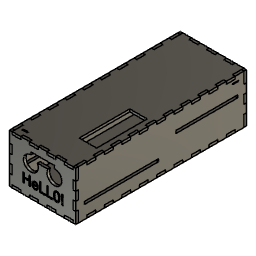
ShellV5 (Autodesk Fusion 360 design; units mm, degrees)
Autodesk Fusion 360 part; units mm, degrees
note: some values were not read from the file. Set by a fixed rule: which sketch regions a step uses.
(part 1 of 2)
sketch "Sketch1" plane through (0, 0, 0) normal (0, 0, 1) x (1, 0, 0)
  line L0 (0, 0) -> (-196, 0)
  line L1 (-196, 0) -> (-196, 76)
  line L2 (-196, 76) -> (0, 76)
  line L3 (0, 76) -> (0, 0)
  dimension "d7" = 196
  dimension "d8" = 76
  constraint horizontal L0
  constraint vertical L1
  constraint horizontal L2
  constraint vertical L3
  constraint coincident L0.start L3.end
  measures "d7" distance of L0.start L0.end
  measures "d8" distance of L0.start L2.end
extrude "Extrude1" add sketch "Sketch1" along normal blind 3 makes body 1
sketch "Sketch2" plane through (0, 0, 0) normal (1, 0, 0) x (0, 1, 0)
  line L0 (76, 0) -> (76, 56)
  line L1 (76, 56) -> (0, 56)
  line L2 (0, 56) -> (0, 0)
  line L3 (0, 56) -> (3, 56)
  line L4 (3, 56) -> (3, 53)
  line L5 (3, 53) -> (0, 53)
  line L6 (0, 53) -> (0, 56)
  line L7 (0, 53) -> (3, 53)
  line L8 (3, 53) -> (3, 43)
  line L9 (3, 43) -> (0, 43)
  line L10 (0, 43) -> (0, 53)
  line L11 (0, 43) -> (3, 43)
  line L12 (3, 43) -> (3, 33)
  line L13 (3, 33) -> (0, 33)
  line L14 (0, 33) -> (0, 43)
  line L15 (0, 33) -> (3, 33)
  line L16 (3, 33) -> (3, 23)
  line L17 (3, 23) -> (0, 23)
  line L18 (0, 23) -> (0, 33)
  line L19 (0, 23) -> (3, 23)
  line L20 (3, 23) -> (3, 13)
  line L21 (3, 13) -> (0, 13)
  line L22 (0, 13) -> (0, 23)
  line L23 (0, 13) -> (3, 13)
  line L24 (3, 13) -> (3, 3)
  line L25 (0, 3) -> (0, 13)
  line L26 (38, 0) -> (38, 56)
  line L27 (76, 13) -> (73, 13)
  line L28 (73, 53) -> (76, 53)
  line L29 (73, 56) -> (73, 53)
  line L30 (73, 23) -> (76, 23)
  line L31 (73, 43) -> (76, 43)
  line L32 (73, 23) -> (73, 13)
  line L33 (73, 13) -> (73, 3)
  line L34 (73, 33) -> (73, 23)
  line L35 (76, 56) -> (73, 56)
  line L36 (73, 53) -> (73, 43)
  line L37 (73, 33) -> (76, 33)
  line L38 (76, 53) -> (73, 53)
  line L39 (73, 13) -> (76, 13)
  line L40 (76, 43) -> (73, 43)
  line L41 (73, 43) -> (73, 33)
  line L42 (76, 23) -> (73, 23)
  line L43 (76, 33) -> (73, 33)
  line L44 (0, 56) -> (38, 56)
  line L45 (0, 56) -> (76, 56)
  line L46 (38, 28) -> (0, 28)
  line L47 (0, 3) -> (3, 3)
  line L48 (3, 3) -> (3, 0)
  line L49 (3, 0) -> (0, 0)
  line L50 (0, 0) -> (0, 3)
  line L51 (3, 3) -> (13, 3)
  line L52 (13, 3) -> (13, 0)
  line L53 (13, 0) -> (3, 0)
  line L54 (3, 0) -> (3, 3)
  line L55 (13, 3) -> (23, 3)
  line L56 (23, 3) -> (23, 0)
  line L57 (23, 0) -> (13, 0)
  line L58 (13, 0) -> (13, 3)
  line L59 (23, 3) -> (33, 3)
  line L60 (33, 3) -> (33, 0)
  line L61 (33, 0) -> (23, 0)
  line L62 (23, 0) -> (23, 3)
  line L63 (33, 3) -> (43, 3)
  line L64 (43, 3) -> (43, 0)
  line L65 (43, 0) -> (33, 0)
  line L66 (33, 0) -> (33, 3)
  line L67 (43, 0) -> (53, 0)
  line L68 (53, 0) -> (53, 3)
  line L69 (53, 3) -> (43, 3)
  line L70 (43, 3) -> (43, 0)
  line L71 (53, 3) -> (63, 3)
  line L72 (63, 3) -> (63, 0)
  line L73 (63, 0) -> (53, 0)
  line L74 (53, 0) -> (53, 3)
  line L75 (63, 3) -> (73, 3)
  line L76 (73, 3) -> (73, 0)
  line L77 (73, 0) -> (63, 0)
  line L78 (63, 0) -> (63, 3)
  line L79 (73, 3) -> (76, 3)
  line L80 (76, 3) -> (76, 0)
  line L81 (76, 0) -> (73, 0)
  line L82 (73, 0) -> (73, 3)
  line L83 (53, 56) -> (53, 53)
  line L84 (3, 53) -> (13, 53)
  line L85 (13, 56) -> (3, 56)
  line L86 (73, 53) -> (73, 56)
  line L87 (13, 56) -> (13, 53)
  line L88 (13, 53) -> (13, 56)
  line L89 (23, 56) -> (13, 56)
  line L90 (0, 53) -> (3, 53)
  line L91 (53, 56) -> (53, 53)
  line L92 (3, 56) -> (3, 53)
  line L93 (23, 56) -> (23, 53)
  line L94 (43, 53) -> (43, 56)
  line L95 (33, 56) -> (33, 53)
  line L96 (43, 53) -> (43, 56)
  line L97 (73, 56) -> (63, 56)
  line L98 (33, 53) -> (33, 56)
  line L99 (23, 53) -> (23, 56)
  line L100 (76, 53) -> (76, 56)
  line L101 (73, 56) -> (73, 53)
  line L102 (3, 53) -> (3, 56)
  line L103 (63, 53) -> (73, 53)
  line L104 (63, 53) -> (63, 56)
  line L105 (53, 53) -> (63, 53)
  line L106 (43, 56) -> (53, 56)
  line L107 (3, 56) -> (0, 56)
  line L108 (23, 53) -> (33, 53)
  line L109 (43, 56) -> (33, 56)
  line L110 (63, 56) -> (63, 53)
  line L111 (33, 56) -> (23, 56)
  line L112 (63, 56) -> (53, 56)
  line L113 (13, 53) -> (23, 53)
  line L114 (0, 56) -> (0, 53)
  line L115 (33, 53) -> (43, 53)
  line L116 (76, 56) -> (73, 56)
  line L117 (53, 53) -> (43, 53)
  line L118 (73, 53) -> (76, 53)
  point P0 (0, 56)
  point P1 (0, 56)
  point P2 (38, 56)
  point P3 (0, 56)
  point P4 (76, 56)
  dimension "d11" = 76
  dimension "d12" = 56
  dimension "d13" = 3
  dimension "d14" = 3
  dimension "d15" = 3
  dimension "d16" = 10
  dimension "d17" = 3
  dimension "d18" = 10
  dimension "d19" = 3
  dimension "d20" = 10
  dimension "d21" = 3
  dimension "d22" = 10
  dimension "d23" = 3
  dimension "d24" = 10
  dimension "d47" = 38
  dimension "d48" = 56
  dimension "d49" = 3
  dimension "d50" = 3
  dimension "d51" = 10
  dimension "d52" = 3
  dimension "d53" = 10
  dimension "d54" = 3
  dimension "d55" = 10
  dimension "d56" = 3
  dimension "d57" = 10
  dimension "d58" = 3
  dimension "d59" = 10
  dimension "d60" = 3
  dimension "d61" = 10
  dimension "d62" = 3
  dimension "d63" = 10
  dimension "d64" = 3
  dimension "d65" = 3
  dimension "d66" = 3
  constraint vertical L0
  constraint horizontal L1
  constraint vertical L2
  constraint coincident L2.end L49.end
  constraint horizontal L3
  constraint vertical L4
  constraint horizontal L5
  constraint vertical L6
  constraint horizontal L7
  constraint vertical L8
  constraint horizontal L9
  constraint vertical L10
  constraint horizontal L11
  constraint vertical L12
  constraint horizontal L13
  constraint vertical L14
  constraint horizontal L15
  constraint vertical L16
  constraint horizontal L17
  constraint vertical L18
  constraint horizontal L19
  constraint vertical L20
  constraint horizontal L21
  constraint vertical L22
  constraint horizontal L23
  constraint vertical L24
  constraint vertical L25
  constraint symmetric P3 L26 L0.end
  constraint symmetric L3.end L26 L29.start
  constraint symmetric L4.end L26 L28.start
  constraint symmetric L5.end L26 L28.end
  constraint symmetric L8.end L26 L31.start
  constraint symmetric L9.end L26 L31.end
  constraint symmetric L12.end L26 L34.start
  constraint symmetric L13.end L26 L37.end
  constraint symmetric L16.end L26 L30.start
  constraint symmetric L17.end L26 L30.end
  constraint symmetric L20.end L26 L27.end
  constraint symmetric L21.end L26 L27.start
  constraint symmetric L24.end L26 L33.end
  constraint midpoint L26 L46.start
  constraint midpoint L18 L46.end
  constraint horizontal L47
  constraint vertical L48
  constraint horizontal L49
  constraint vertical L50
  constraint horizontal L51
  constraint vertical L52
  constraint horizontal L53
  constraint vertical L54
  constraint horizontal L55
  constraint vertical L56
  constraint horizontal L57
  constraint vertical L58
  constraint horizontal L59
  constraint vertical L60
  constraint horizontal L61
  constraint vertical L62
  constraint horizontal L63
  constraint vertical L64
  constraint horizontal L65
  constraint vertical L66
  constraint horizontal L67
  constraint vertical L68
  constraint horizontal L69
  constraint vertical L70
  constraint horizontal L71
  constraint vertical L72
  constraint horizontal L73
  constraint vertical L74
  constraint horizontal L75
  constraint vertical L76
  constraint horizontal L77
  constraint vertical L78
  constraint horizontal L79
  constraint vertical L80
  constraint horizontal L81
  constraint vertical L82
  constraint symmetric L2.end L46 P3
  constraint symmetric L0.start L46 P4
  constraint symmetric L24.end L46 L4.end
  constraint symmetric L25.start L46 L5.end
  constraint symmetric L26.start L46 P2
  constraint symmetric L33.end L46 L28.start
  constraint symmetric L46 L24.end L4.end
  constraint symmetric L46 L48.end L3.end
  constraint symmetric L46 L2.end P3
  constraint symmetric L46 L51.end L84.end
  constraint symmetric L46 L52.end L85.start
  constraint symmetric L46 L55.end L93.end
  constraint symmetric L46 L56.end L89.start
  constraint symmetric L46 L59.end L95.end
  constraint symmetric L46 L60.end L95.start
  constraint symmetric L46 L63.end L94.start
  constraint symmetric L46 L64.end L94.end
  constraint symmetric L46 L67.end L83.start
  constraint symmetric L46 L68.end L83.end
  constraint symmetric L46 L71.end L103.start
  constraint symmetric L46 L72.end L97.end
  constraint symmetric L46 L33.end L28.start
  constraint symmetric L46 L76.end L29.start
  constraint symmetric L46 L79.end L28.end
  constraint symmetric L46 L0.start P4
  measures "d11" distance of L2.end L0.start
  measures "d12" distance of L2.end P3
  measures "d13" distance of P3 L3.end
  measures "d14" distance of P3 L5.end
  measures "d15" distance of L5.end L4.end
  measures "d16" distance of L5.end L9.end
  measures "d17" distance of L9.end L8.end
  measures "d18" distance of L9.end L13.end
  measures "d19" distance of L13.end L12.end
  measures "d20" distance of L13.end L17.end
  measures "d21" distance of L17.end L16.end
  measures "d22" distance of L17.end L21.end
  measures "d23" distance of L21.end L20.end
  measures "d24" distance of L21.end L25.start
  measures "d47" distance of L2.end L26.start
  measures "d48" distance of L26.start P2
  measures "d49" distance of L25.start L24.end
  measures "d50" distance of L25.start L2.end
  measures "d51" distance of L24.end L51.end
  measures "d52" distance of L24.end L48.end
  measures "d53" distance of L51.end L55.end
  measures "d54" distance of L51.end L52.end
  measures "d55" distance of L55.end L59.end
  measures "d56" distance of L55.end L56.end
  measures "d57" distance of L59.end L63.end
  measures "d58" distance of L59.end L60.end
  measures "d59" distance of L64.end L67.end
  measures "d60" distance of L64.end L63.end
  measures "d61" distance of L68.end L71.end
  measures "d62" distance of L68.end L67.end
  measures "d63" distance of L71.end L33.end
  measures "d64" distance of L71.end L72.end
  measures "d65" distance of L33.end L79.end
  measures "d66" distance of L33.end L76.end
extrude "Extrude2" add sketch "Sketch2" against normal blind 3 separate body contours L0 L76 L79 L80 L81 L82 | L0 L27 L33 L39 L79 | L26 L32 L33 L34 L36 L41 L63 L69 L71 L75 L103 L105 L115 L117 | L68 L71 L72 L73 L74 L78 | L0 L30 L34 L37 L42 L43 | L26 L63 L64 L65 L70 | L0 L28 L31 L36 L38 L40 L118 | L26 L60 L63 L65 L66 | L0 L1 L28 L29 L35 L38 L45 L86 L100 L101 L116 L118 | L16 L20 L24 L26 L46 L51 L55 L59 L63 | L8 L12 L16 L26 L46 L84 L108 L113 L115 | L52 L55 L56 L57 L58 L62 | L1 L45 L83 L91 L104 L105 L110 L112 | L1 L26 L44 L45 L95 L98 L109 L115 | L1 L26 L45 L94 L96 L109 L115 | L2 L13 L15 L16 L18 L46 | L2 L16 L17 L18 L19 L46 | L2 L47 L48 L49 L50 L54 | L1 L44 L45 L87 L88 L89 L93 L99 L113 | L2 L5 L7 L8 L9 L10 L11 L90 | L2 L21 L23 L24 L25 L47 | L1 L2 L3 L4 L5 L6 L7 L44 L45 L90 L92 L102 L107 L114 makes body 2
combine "Combine1" operation cut target body 1 tool bodies 2 keep tools
sketch "Sketch3" plane through (0, 76, 0) normal (0, 1, 0) x (-1, 0, 0)
  line L0 (3, 3) -> (3, 0)
  line L1 (3, 0) -> (196, 0)
  line L2 (196, 0) -> (196, 3)
  line L3 (196, 3) -> (3, 3)
  line L4 (0, 0) -> (196, 0)
  line L5 (196, 0) -> (196, 56)
  line L6 (196, 56) -> (0, 56)
  line L7 (0, 56) -> (0, 0)
  line L8 (0, 56) -> (3, 56)
  line L9 (3, 56) -> (3, 53)
  line L10 (3, 53) -> (0, 53)
  line L11 (0, 53) -> (0, 56)
  line L12 (0, 53) -> (3, 53)
  line L13 (3, 53) -> (3, 43)
  line L14 (3, 43) -> (0, 43)
  line L15 (0, 43) -> (0, 53)
  line L16 (0, 43) -> (3, 43)
  line L17 (3, 43) -> (3, 33)
  line L18 (3, 33) -> (0, 33)
  line L19 (0, 33) -> (0, 43)
  line L20 (0, 0) -> (3, 0)
  line L21 (3, 0) -> (3, 3)
  line L22 (3, 3) -> (0, 3)
  line L23 (0, 3) -> (0, 0)
  line L24 (0, 3) -> (3, 3)
  line L25 (3, 3) -> (3, 13)
  line L26 (3, 13) -> (0, 13)
  line L27 (0, 13) -> (0, 3)
  line L28 (0, 13) -> (3, 13)
  line L29 (3, 13) -> (3, 23)
  line L30 (3, 23) -> (0, 23)
  line L31 (0, 23) -> (0, 13)
  line L32 (3, 3) -> (13, 3)
  line L33 (13, 3) -> (13, 0)
  line L34 (13, 0) -> (3, 0)
  line L35 (3, 0) -> (3, 3)
  line L36 (13, 0) -> (23, 0)
  line L37 (23, 0) -> (23, 3)
  line L38 (23, 3) -> (13, 3)
  line L39 (13, 3) -> (13, 0)
  line L40 (23, 0) -> (33, 0)
  line L41 (33, 0) -> (33, 3)
  line L42 (33, 3) -> (23, 3)
  line L43 (23, 3) -> (23, 0)
  line L44 (33, 0) -> (43, 0)
  line L45 (43, 0) -> (43, 3)
  line L46 (43, 3) -> (33, 3)
  line L47 (33, 3) -> (33, 0)
  line L48 (43, 0) -> (53, 0)
  line L49 (53, 0) -> (53, 3)
  line L50 (53, 3) -> (43, 3)
  line L51 (43, 3) -> (43, 0)
  line L52 (53, 0) -> (63, 0)
  line L53 (63, 0) -> (63, 3)
  line L54 (63, 3) -> (53, 3)
  line L55 (53, 3) -> (53, 0)
  line L56 (63, 0) -> (73, 0)
  line L57 (73, 0) -> (73, 3)
  line L58 (73, 3) -> (63, 3)
  line L59 (63, 3) -> (63, 0)
  line L60 (73, 0) -> (83, 0)
  line L61 (83, 0) -> (83, 3)
  line L62 (83, 3) -> (73, 3)
  line L63 (73, 3) -> (73, 0)
  line L64 (83, 0) -> (93, 0)
  line L65 (93, 0) -> (93, 3)
  line L66 (93, 3) -> (83, 3)
  line L67 (83, 3) -> (83, 0)
  line L68 (93, 0) -> (103, 0)
  line L69 (103, 0) -> (103, 3)
  line L70 (103, 3) -> (93, 3)
  line L71 (93, 3) -> (93, 0)
  line L72 (103, 0) -> (113, 0)
  line L73 (113, 0) -> (113, 3)
  line L74 (113, 3) -> (103, 3)
  line L75 (103, 3) -> (103, 0)
  line L76 (113, 0) -> (123, 0)
  line L77 (123, 0) -> (123, 3)
  line L78 (123, 3) -> (113, 3)
  line L79 (113, 3) -> (113, 0)
  line L80 (123, 0) -> (133, 0)
  line L81 (133, 0) -> (133, 3)
  line L82 (133, 3) -> (123, 3)
  line L83 (123, 3) -> (123, 0)
  line L84 (133, 0) -> (143, 0)
  line L85 (143, 0) -> (143, 3)
  line L86 (143, 3) -> (133, 3)
  line L87 (133, 3) -> (133, 0)
  line L88 (143, 0) -> (153, 0)
  line L89 (153, 0) -> (153, 3)
  line L90 (153, 3) -> (143, 3)
  line L91 (143, 3) -> (143, 0)
  line L92 (153, 0) -> (163, 0)
  line L93 (163, 0) -> (163, 3)
  line L94 (163, 3) -> (153, 3)
  line L95 (153, 3) -> (153, 0)
  line L96 (163, 3) -> (173, 3)
  line L97 (173, 3) -> (173, 0)
  line L98 (173, 0) -> (163, 0)
  line L99 (163, 0) -> (163, 3)
  line L100 (173, 3) -> (183, 3)
  line L101 (183, 3) -> (183, 0)
  line L102 (183, 0) -> (173, 0)
  line L103 (173, 0) -> (173, 3)
  line L104 (183, 3) -> (193, 3)
  line L105 (193, 3) -> (193, 0)
  line L106 (193, 0) -> (183, 0)
  line L107 (183, 0) -> (183, 3)
  line L108 (193, 3) -> (196, 3)
  line L109 (196, 3) -> (196, 0)
  line L110 (196, 0) -> (193, 0)
  line L111 (193, 0) -> (193, 3)
  line L112 (0, 0) -> (78, 0)
  line L113 (0, 0) -> (88, 0)
  line L114 (88, 28) -> (196, 28)
  line L115 (3, 53) -> (3, 56)
  line L116 (153, 56) -> (163, 56)
  line L117 (163, 56) -> (163, 53)
  line L118 (133, 53) -> (133, 56)
  line L119 (133, 53) -> (123, 53)
  line L120 (173, 53) -> (183, 53)
  line L121 (193, 56) -> (193, 53)
  line L122 (3, 56) -> (196, 56)
  line L123 (196, 53) -> (3, 53)
  line L124 (196, 53) -> (196, 56)
  line L125 (173, 56) -> (173, 53)
  line L126 (143, 53) -> (133, 53)
  line L127 (183, 56) -> (183, 53)
  line L128 (193, 53) -> (196, 53)
  line L129 (196, 56) -> (196, 53)
  line L130 (193, 53) -> (193, 56)
  line L131 (183, 53) -> (193, 53)
  line L132 (123, 56) -> (133, 56)
  line L133 (153, 56) -> (153, 53)
  line L134 (33, 53) -> (33, 56)
  line L135 (173, 53) -> (173, 56)
  line L136 (0, 56) -> (196, 56)
  line L137 (163, 53) -> (173, 53)
  line L138 (163, 56) -> (163, 53)
  line L139 (53, 56) -> (53, 53)
  line L140 (93, 53) -> (93, 56)
  line L141 (183, 53) -> (183, 56)
  line L142 (143, 56) -> (153, 56)
  line L143 (113, 56) -> (123, 56)
  line L144 (183, 56) -> (173, 56)
  line L145 (103, 56) -> (113, 56)
  line L146 (143, 53) -> (143, 56)
  line L147 (196, 56) -> (193, 56)
  line L148 (0, 56) -> (78, 56)
  line L149 (63, 56) -> (73, 56)
  line L150 (0, 56) -> (88, 56)
  line L151 (133, 56) -> (133, 53)
  line L152 (73, 53) -> (63, 53)
  line L153 (13, 56) -> (3, 56)
  line L154 (83, 56) -> (83, 53)
  line L155 (153, 53) -> (143, 53)
  line L156 (133, 56) -> (143, 56)
  line L157 (0, 53) -> (3, 53)
  line L158 (123, 53) -> (113, 53)
  line L159 (93, 56) -> (93, 53)
  line L160 (103, 53) -> (93, 53)
  line L161 (73, 56) -> (83, 56)
  line L162 (13, 56) -> (23, 56)
  line L163 (153, 53) -> (153, 56)
  line L164 (83, 53) -> (83, 56)
  line L165 (163, 53) -> (153, 53)
  line L166 (143, 56) -> (143, 53)
  line L167 (13, 53) -> (13, 56)
  line L168 (123, 56) -> (123, 53)
  line L169 (173, 56) -> (163, 56)
  line L170 (53, 53) -> (43, 53)
  line L171 (83, 56) -> (93, 56)
  line L172 (43, 53) -> (33, 53)
  line L173 (103, 53) -> (103, 56)
  line L174 (193, 56) -> (183, 56)
  line L175 (113, 56) -> (113, 53)
  line L176 (33, 56) -> (33, 53)
  line L177 (23, 56) -> (33, 56)
  line L178 (113, 53) -> (103, 53)
  line L179 (0, 56) -> (3, 56)
  line L180 (23, 53) -> (23, 56)
  line L181 (73, 53) -> (73, 56)
  line L182 (103, 56) -> (103, 53)
  line L183 (93, 56) -> (103, 56)
  line L184 (3, 53) -> (13, 53)
  line L185 (73, 56) -> (73, 53)
  line L186 (63, 56) -> (63, 53)
  line L187 (3, 56) -> (3, 53)
  line L188 (53, 56) -> (63, 56)
  line L189 (33, 56) -> (43, 56)
  line L190 (113, 53) -> (113, 56)
  line L191 (53, 53) -> (53, 56)
  line L192 (43, 53) -> (43, 56)
  line L193 (63, 53) -> (53, 53)
  line L194 (63, 53) -> (63, 56)
  line L195 (123, 53) -> (123, 56)
  line L196 (93, 53) -> (83, 53)
  line L197 (33, 53) -> (23, 53)
  line L198 (13, 53) -> (13, 56)
  line L199 (43, 56) -> (53, 56)
  line L200 (0, 53) -> (0, 56)
  line L201 (83, 53) -> (73, 53)
  line L202 (23, 53) -> (13, 53)
  line L203 (3, 56) -> (3, 53)
  line L204 (43, 56) -> (43, 53)
  line L205 (23, 56) -> (23, 53)
  line L206 (3, 53) -> (0, 53)
  line L207 (196, 0) -> (98, 0)
  line L208 (98, 0) -> (98, 53)
  line L209 (0, 33) -> (3, 33)
  line L210 (3, 33) -> (3, 23)
  line L211 (3, 23) -> (0, 23)
  line L212 (0, 23) -> (0, 33)
  line L213 (193, 53) -> (193, 56)
  line L214 (196, 3) -> (193, 3)
  line L215 (193, 3) -> (196, 3)
  line L216 (193, 43) -> (193, 33)
  line L217 (196, 3) -> (196, 0)
  line L218 (193, 56) -> (193, 53)
  line L219 (193, 56) -> (193, 53)
  line L220 (196, 33) -> (196, 43)
  line L221 (196, 33) -> (193, 33)
  line L222 (193, 56) -> (193, 53)
  line L223 (196, 56) -> (193, 56)
  line L224 (196, 56) -> (193, 56)
  line L225 (196, 43) -> (193, 43)
  line L226 (196, 53) -> (196, 56)
  line L227 (196, 13) -> (193, 13)
  line L228 (193, 13) -> (196, 13)
  line L229 (193, 23) -> (196, 23)
  line L230 (196, 13) -> (196, 3)
  line L231 (193, 43) -> (196, 43)
  line L232 (196, 53) -> (196, 56)
  line L233 (196, 53) -> (193, 53)
  line L234 (196, 23) -> (196, 33)
  line L235 (196, 53) -> (193, 53)
  line L236 (193, 23) -> (196, 23)
  line L237 (196, 56) -> (196, 0)
  line L238 (193, 3) -> (193, 13)
  line L239 (193, 53) -> (196, 53)
  line L240 (193, 3) -> (193, 0)
  line L241 (193, 33) -> (193, 23)
  line L242 (193, 53) -> (193, 43)
  line L243 (193, 33) -> (196, 33)
  line L244 (196, 43) -> (196, 53)
  line L245 (196, 23) -> (196, 13)
  line L246 (193, 0) -> (193, 3)
  line L247 (196, 0) -> (193, 0)
  line L248 (193, 0) -> (193, 3)
  line L249 (193, 53) -> (196, 53)
  line L250 (193, 13) -> (193, 23)
  point P0 (0, 56)
  point P1 (196, 56)
  point P2 (196, 0)
  point P3 (196, 56)
  dimension "d69" = 196
  dimension "d70" = 56
  dimension "d71" = 3
  dimension "d72" = 3
  dimension "d73" = 3
  dimension "d74" = 10
  dimension "d75" = 3
  dimension "d76" = 10
  dimension "d77" = 3
  dimension "d78" = 3
  dimension "d79" = 3
  dimension "d80" = 10
  dimension "d81" = 3
  dimension "d82" = 10
  dimension "d83" = 10
  dimension "d84" = 3
  dimension "d85" = 10
  dimension "d86" = 3
  dimension "d87" = 10
  dimension "d88" = 3
  dimension "d89" = 10
  dimension "d90" = 3
  dimension "d91" = 10
  dimension "d92" = 3
  dimension "d93" = 10
  dimension "d94" = 3
  dimension "d95" = 10
  dimension "d96" = 3
  dimension "d97" = 10
  dimension "d98" = 3
  dimension "d99" = 10
  dimension "d100" = 3
  dimension "d101" = 10
  dimension "d102" = 3
  dimension "d103" = 10
  dimension "d104" = 10
  dimension "d105" = 3
  dimension "d106" = 10
  dimension "d107" = 3
  dimension "d108" = 10
  dimension "d109" = 3
  dimension "d110" = 10
  dimension "d111" = 3
  dimension "d112" = 10
  dimension "d113" = 3
  dimension "d114" = 10
  dimension "d115" = 3
  dimension "d116" = 10
  dimension "d117" = 3
  dimension "d118" = 10
  dimension "d119" = 3
  dimension "d120" = 3
  dimension "d121" = 3
  dimension "d122" = 98
  dimension "d123" = 3
  dimension "d124" = 10
  constraint horizontal L4
  constraint vertical L5
  constraint horizontal L6
  constraint vertical L7
  constraint coincident L4.start L7.end
  constraint horizontal L8
  constraint vertical L9
  constraint horizontal L10
  constraint vertical L11
  constraint horizontal L12
  constraint vertical L13
  constraint horizontal L14
  constraint vertical L15
  constraint horizontal L16
  constraint vertical L17
  constraint horizontal L18
  constraint vertical L19
  constraint horizontal L20
  constraint vertical L21
  constraint horizontal L22
  constraint vertical L23
  constraint horizontal L24
  constraint vertical L25
  constraint horizontal L26
  constraint vertical L27
  constraint horizontal L28
  constraint vertical L29
  constraint horizontal L30
  constraint vertical L31
  constraint horizontal L32
  constraint vertical L33
  constraint horizontal L34
  constraint vertical L35
  constraint horizontal L36
  constraint vertical L37
  constraint horizontal L38
  constraint vertical L39
  constraint horizontal L40
  constraint vertical L41
  constraint horizontal L42
  constraint vertical L43
  constraint horizontal L44
  constraint vertical L45
  constraint horizontal L46
  constraint vertical L47
  constraint horizontal L48
  constraint vertical L49
  constraint horizontal L50
  constraint vertical L51
  constraint horizontal L52
  constraint vertical L53
  constraint horizontal L54
  constraint vertical L55
  constraint horizontal L56
  constraint vertical L57
  constraint horizontal L58
  constraint vertical L59
  constraint horizontal L60
  constraint vertical L61
  constraint horizontal L62
  constraint vertical L63
  constraint horizontal L64
  constraint vertical L65
  constraint horizontal L66
  constraint vertical L67
  constraint horizontal L68
  constraint vertical L69
  constraint horizontal L70
  constraint vertical L71
  constraint horizontal L72
  constraint vertical L73
  constraint horizontal L74
  constraint vertical L75
  constraint horizontal L76
  constraint vertical L77
  constraint horizontal L78
  constraint vertical L79
  constraint horizontal L80
  constraint vertical L81
  constraint horizontal L82
  constraint vertical L83
  constraint horizontal L84
  constraint vertical L85
  constraint horizontal L86
  constraint vertical L87
  constraint horizontal L88
  constraint vertical L89
  constraint horizontal L90
  constraint vertical L91
  constraint horizontal L92
  constraint vertical L93
  constraint horizontal L94
  constraint vertical L95
  constraint horizontal L96
  constraint vertical L97
  constraint horizontal L98
  constraint vertical L99
  constraint horizontal L100
  constraint vertical L101
  constraint horizontal L102
  constraint vertical L103
  constraint horizontal L104
  constraint vertical L105
  constraint horizontal L106
  constraint vertical L107
  constraint horizontal L108
  constraint vertical L109
  constraint horizontal L110
  constraint vertical L111
  constraint midpoint L60 L112.end
  constraint midpoint L64 L113.end
  constraint midpoint L5 L114.end
  constraint symmetric L4.start L114 L6.end
  constraint symmetric L0.start L114 L9.end
  constraint symmetric L0.end L114 L8.end
  constraint symmetric P2 L114 P1
  constraint symmetric L2.end L114 L123.start
  constraint symmetric L4.start L114 P0
  constraint symmetric P2 L114 P3
  constraint symmetric L22.end L114 L10.end
  constraint symmetric L32.end L114 L167.start
  constraint symmetric L33.end L114 L153.start
  constraint symmetric L36.end L114 L162.end
  constraint symmetric L37.end L114 L180.start
  constraint symmetric L40.end L114 L134.end
  constraint symmetric L41.end L114 L134.start
  constraint symmetric L44.end L114 L189.end
  constraint symmetric L45.end L114 L170.end
  constraint symmetric L48.end L114 L139.start
  constraint symmetric L49.end L114 L139.end
  constraint symmetric L52.end L114 L149.start
  constraint symmetric L53.end L114 L152.end
  constraint symmetric L56.end L114 L149.end
  constraint symmetric L57.end L114 L152.start
  constraint symmetric L60.end L114 L154.start
  constraint symmetric L61.end L114 L154.end
  constraint symmetric L64.end L114 L140.end
  constraint symmetric L65.end L114 L140.start
  constraint symmetric L68.end L114 L145.start
  constraint symmetric L69.end L114 L160.start
  constraint symmetric L72.end L114 L143.start
  constraint symmetric L73.end L114 L158.end
  constraint symmetric L76.end L114 L132.start
  constraint symmetric L77.end L114 L119.end
  constraint symmetric L80.end L114 L118.end
  constraint symmetric L81.end L114 L118.start
  constraint symmetric L84.end L114 L142.start
  constraint symmetric L85.end L114 L126.start
  constraint symmetric L88.end L114 L116.start
  constraint symmetric L89.end L114 L133.end
  constraint symmetric L92.end L114 L116.end
  constraint symmetric L93.end L114 L117.end
  constraint symmetric L96.end L114 L120.start
  constraint symmetric L97.end L114 L125.start
  constraint symmetric L100.end L114 L120.end
  constraint symmetric L101.end L114 L127.start
  constraint symmetric L104.end L114 L121.end
  constraint symmetric L105.end L114 L121.start
  constraint symmetric L112.end L114 L148.end
  constraint symmetric L113.end L114 L150.end
  constraint coincident P2 L1.end
  constraint perpendicular L99 L207
  constraint midpoint L160 L208.end
  constraint perpendicular L123 L208
  constraint horizontal L209
  constraint vertical L210
  constraint horizontal L211
  constraint vertical L212
  constraint symmetric L4.start L208 P2
  constraint symmetric L0.start L208 L104.end
  constraint symmetric L0.end L208 L105.end
  constraint symmetric P0 L208 P3
  constraint symmetric L8.end L208 L121.start
  constraint symmetric L9.end L208 L121.end
  constraint symmetric L10.end L208 L123.start
  constraint symmetric L13.end L208 L216.start
  constraint symmetric L14.end L208 L220.end
  constraint symmetric L17.end L208 L216.end
  constraint symmetric L18.end L208 L220.start
  constraint symmetric L22.end L208 L2.end
  constraint symmetric L25.end L208 L227.end
  constraint symmetric L26.end L208 L227.start
  constraint symmetric L29.end L208 L229.start
  constraint symmetric L30.end L208 L229.end
  constraint symmetric L208 L17.end L216.end
  constraint symmetric L208 L29.end L229.start
  constraint symmetric L208 L30.end L229.end
  measures "d69" distance of L4.start P2
  measures "d70" distance of L4.start P0
  measures "d71" distance of P0 L8.end
  measures "d72" distance of P0 L10.end
  measures "d73" distance of L10.end L9.end
  measures "d74" distance of L10.end L14.end
  measures "d75" distance of L14.end L13.end
  measures "d76" distance of L14.end L18.end
  measures "d77" distance of L4.start L0.end
  measures "d78" distance of L4.start L22.end
  measures "d79" distance of L22.end L0.start
  measures "d80" distance of L22.end L26.end
  measures "d81" distance of L26.end L25.end
  measures "d82" distance of L26.end L30.end
  measures "d83" distance of L0.start L32.end
  measures "d84" distance of L0.start L0.end
  measures "d85" distance of L33.end L36.end
  measures "d86" distance of L33.end L32.end
  measures "d87" distance of L36.end L40.end
  measures "d88" distance of L36.end L37.end
  measures "d89" distance of L40.end L44.end
  measures "d90" distance of L40.end L41.end
  measures "d91" distance of L44.end L48.end
  measures "d92" distance of L44.end L45.end
  measures "d93" distance of L48.end L52.end
  measures "d94" distance of L48.end L49.end
  measures "d95" distance of L52.end L56.end
  measures "d96" distance of L52.end L53.end
  measures "d97" distance of L56.end L60.end
  measures "d98" distance of L56.end L57.end
  measures "d99" distance of L60.end L64.end
  measures "d100" distance of L60.end L61.end
  measures "d101" distance of L64.end L68.end
  measures "d102" distance of L64.end L65.end
  measures "d103" distance of L68.end L72.end
  measures "d104" distance of L72.end L76.end
  measures "d105" distance of L72.end L73.end
  measures "d106" distance of L76.end L80.end
  measures "d107" distance of L76.end L77.end
  measures "d108" distance of L80.end L84.end
  measures "d109" distance of L80.end L81.end
  measures "d110" distance of L84.end L88.end
  measures "d111" distance of L84.end L85.end
  measures "d112" distance of L88.end L92.end
  measures "d113" distance of L88.end L89.end
  measures "d114" distance of L93.end L96.end
  measures "d115" distance of L93.end L92.end
  measures "d116" distance of L96.end L100.end
  measures "d117" distance of L96.end L97.end
  measures "d118" distance of L100.end L104.end
  measures "d119" distance of L100.end L101.end
  measures "d120" distance of L104.end L2.end
  measures "d121" distance of L104.end L105.end
  measures "d122" distance of P2 L207.end
  measures "d123" distance of L18.end L17.end
  measures "d124" distance of L18.end L30.end
extrude "Extrude3" add sketch "Sketch3" against normal blind 3 separate body contours L0 L1 L3 L4 L21 L32 L33 L34 L35 L39 L112 L113 | L3 L13 L17 L25 L29 L32 L38 L42 L46 L50 L54 L58 L62 L66 L70 L123 L152 L160 L170 L172 L184 L193 L196 L197 L201 L202 L208 L210 | L7 L26 L28 L29 L30 L31 L211 | L1 L3 L4 L37 L40 L41 L42 L43 L47 L112 L113 | L7 L14 L16 L17 L18 L19 L209 | L1 L3 L4 L45 L48 L49 L50 L51 L55 L112 L113 | L6 L9 L115 L122 L123 L136 L148 L150 L153 L167 L184 L187 L198 L203 | L1 L3 L4 L53 L56 L57 L58 L59 L63 L112 L113 | L6 L122 L123 L134 L136 L148 L150 L176 L177 L180 L197 L205 | L1 L3 L4 L61 L64 L65 L66 L67 L71 L113 | L6 L122 L123 L136 L139 L148 L150 L170 L191 L192 L199 L204 | L3 L70 L74 L78 L82 L86 L90 L94 L96 L100 L104 L114 L208 L238 L241 L250 | L1 L3 L4 L69 L72 L73 L74 L75 L79 L207 | L114 L119 L120 L123 L126 L131 L137 L155 L158 L160 L165 L178 L208 L216 L241 L242 | L6 L122 L123 L136 L148 L149 L150 L152 L181 L185 L186 L194 | L1 L3 L4 L77 L80 L81 L82 L83 L87 L207 | L5 L216 L220 L221 L225 L231 L237 L243 | L5 L227 L228 L229 L236 L237 L245 L250 | L6 L122 L123 L136 L145 L173 L175 L178 L182 L190 | L6 L122 L123 L136 L140 L150 L154 L159 L164 L171 L196 | L1 L3 L4 L85 L88 L89 L90 L91 L95 L207 | L6 L121 L122 L123 L127 L130 L131 L136 L141 L174 L213 L218 L219 L222 | L1 L3 L4 L101 L104 L105 L106 L107 L111 L207 L240 L246 L248 | L6 L118 L119 L122 L123 L132 L136 L151 L168 L195 | L1 L3 L4 L93 L96 L97 L98 L99 L103 L207 | L6 L117 L122 L123 L125 L135 L136 L137 L138 L169 | L6 L122 L123 L133 L136 L142 L146 L155 L163 L166 makes body 3
combine "Combine2" operation cut target body 1 tool bodies 3 keep tools
ref_plane "WorkPlane1" through (-98, 38, 28) normal (1, 0, 0) x (0, 1, 0)
mirror "Mirror1" about plane through (-98, 38, 28) normal (1, 0, 0) of bodies 2 makes body 4
combine "Combine3" operation cut target body 1 tool bodies 4 keep tools
ref_plane "WorkPlane2" through (-98, 38, 28) normal (0, 1, 0) x (-1, 0, 0)
mirror "Mirror2" about plane through (-98, 38, 28) normal (0, 1, 0) of bodies 3 makes body 5
combine "Combine4" operation cut target body 1 tool bodies 5 keep tools
ref_plane "WorkPlane3" through (-98, 38, 28) normal (0, 0, -1) x (-1, 0, 0)
mirror "Mirror3" about plane through (-98, 38, 28) normal (0, 0, -1) of bodies 1 makes body 6
sketch "Sketch4" plane through (0, 0, 0) normal (1, 0, 0) x (0, 1, 0)
  line L0 (63, 56) -> (53, 56)
  line L1 (53, 56) -> (53, 53)
  line L2 (53, 53) -> (43, 53)
  line L3 (43, 53) -> (43, 56)
  line L4 (43, 56) -> (33, 56)
  line L5 (33, 56) -> (33, 53)
  line L6 (33, 53) -> (23, 53)
  line L7 (23, 53) -> (23, 56)
  line L8 (23, 56) -> (13, 56)
  line L9 (13, 56) -> (13, 53)
  line L10 (13, 53) -> (3, 53)
  line L11 (3, 53) -> (3, 56)
  line L12 (3, 56) -> (0, 56)
  line L13 (0, 56) -> (0, 43)
  line L14 (0, 43) -> (3, 43)
  line L15 (3, 43) -> (3, 33)
  line L16 (3, 33) -> (0, 33)
  line L17 (0, 33) -> (0, 23)
  line L18 (0, 23) -> (3, 23)
  line L19 (3, 23) -> (3, 13)
  line L20 (3, 13) -> (0, 13)
  line L21 (0, 13) -> (0, 0)
  line L22 (0, 0) -> (3, 0)
  line L23 (3, 0) -> (3, 3)
  line L24 (3, 3) -> (13, 3)
  line L25 (13, 3) -> (13, 0)
  line L26 (13, 0) -> (23, 0)
  line L27 (23, 0) -> (23, 3)
  line L28 (23, 3) -> (33, 3)
  line L29 (33, 3) -> (33, 0)
  line L30 (33, 0) -> (43, 0)
  line L31 (43, 0) -> (43, 3)
  line L32 (43, 3) -> (53, 3)
  line L33 (53, 3) -> (53, 0)
  line L34 (53, 0) -> (63, 0)
  line L35 (63, 0) -> (63, 3)
  line L36 (63, 3) -> (73, 3)
  line L37 (73, 3) -> (73, 0)
  line L38 (73, 0) -> (76, 0)
  line L39 (76, 0) -> (76, 13)
  line L40 (76, 13) -> (73, 13)
  line L41 (73, 13) -> (73, 23)
  line L42 (73, 23) -> (76, 23)
  line L43 (76, 23) -> (76, 33)
  line L44 (76, 33) -> (73, 33)
  line L45 (73, 33) -> (73, 43)
  line L46 (73, 43) -> (76, 43)
  line L47 (76, 43) -> (76, 56)
  line L48 (76, 56) -> (73, 56)
  line L49 (73, 56) -> (73, 53)
  line L50 (73, 53) -> (63, 53)
  line L51 (63, 53) -> (63, 56)
  line L52 (0, 0) -> (38, 0)
  line L53 (38, 0) -> (38, 35)
  line L54 (38, 35) -> (33, 35)
  circle A0 centre (24.5, 35) radius 8.5
  line L55 (38, 35) -> (43, 35)
  circle A1 centre (51.5, 35) radius 8.5
  line L56 (24.5, 35) -> (24.5, 43.5)
  line L57 (24.5, 43.5) -> (24.5, 46.5)
  line L58 (24.5, 43.5) -> (51.5, 43.5)
  line L59 (51.5, 43.5) -> (51.5, 46.5)
  line L60 (24.5, 46.5) -> (51.5, 46.5)
  line L61 (31.9375, 39.115) -> (44.0625, 39.115)
  dimension "d133" = 38
  dimension "d134" = 35
  dimension "d135" = 5
  dimension "d136" = 17
  dimension "d137" = 5
  dimension "d138" = 17
  dimension "d139" = 3
  dimension "d140" = 3
  constraint coincident L21.end L22.start
  constraint perpendicular L23 L52
  constraint perpendicular L52 L53
  constraint perpendicular L53 L54
  constraint coincident L54.end A0
  constraint perpendicular L53 L55
  constraint coincident L55.end A1
  constraint coincident A0.centre L56.start
  constraint coincident A0 L56.end
  constraint vertical L56
  constraint parallel L56 L57
  constraint coincident A1 L58.end
  constraint tangent A1 L58
  constraint perpendicular L56 L58
  constraint perpendicular L58 L59
  constraint coincident A0 L61.start
  constraint coincident A1 L61.end
  constraint parallel L58 L61
  measures "d133" distance of L21.end L52.end
  measures "d134" distance of L52.end L53.end
  measures "d135" distance of L53.end L54.end
  measures "d136" diameter of A0
  measures "d137" distance of L53.end L55.end
  measures "d138" diameter of A1
  measures "d139" distance of L56.end L57.end
  measures "d140" distance of L58.end L59.end
extrude "Extrude4" cut sketch "Sketch4" against normal blind 3 contours A0 | A1 | A0 A1 L58 L61 | L57 L58 L59 L60 bodies 2
sketch "Sketch5" plane through (0, 0, 0) normal (1, 0, 0) x (0, 1, 0)
  line L0 (24.5, 46.5) -> (51.5, 46.5)
  line L1 (51.5, 46.5) -> (51.5, 43.5)
  arc A0 (44.0625, 39.115) -> (51.5, 43.5) centre (51.5, 35) ccw
  line L2 (44.0625, 39.115) -> (31.9375, 39.115)
  arc A1 (24.5, 43.5) -> (31.9375, 39.115) centre (24.5, 35) ccw
  line L3 (24.5, 43.5) -> (24.5, 46.5)
  line L4 (63, 56) -> (53, 56)
  line L5 (53, 56) -> (53, 53)
  line L6 (53, 53) -> (43, 53)
  line L7 (43, 53) -> (43, 56)
  line L8 (43, 56) -> (33, 56)
  line L9 (33, 56) -> (33, 53)
  line L10 (33, 53) -> (23, 53)
  line L11 (23, 53) -> (23, 56)
  line L12 (23, 56) -> (13, 56)
  line L13 (13, 56) -> (13, 53)
  line L14 (13, 53) -> (3, 53)
  line L15 (3, 53) -> (3, 56)
  line L16 (3, 56) -> (0, 56)
  line L17 (0, 56) -> (0, 43)
  line L18 (0, 43) -> (3, 43)
  line L19 (3, 43) -> (3, 33)
  line L20 (3, 33) -> (0, 33)
  line L21 (0, 33) -> (0, 23)
  line L22 (0, 23) -> (3, 23)
  line L23 (3, 23) -> (3, 13)
  line L24 (3, 13) -> (0, 13)
  line L25 (0, 13) -> (0, 0)
  line L26 (0, 0) -> (3, 0)
  line L27 (3, 0) -> (3, 3)
  line L28 (3, 3) -> (13, 3)
  line L29 (13, 3) -> (13, 0)
  line L30 (13, 0) -> (23, 0)
  line L31 (23, 0) -> (23, 3)
  line L32 (23, 3) -> (33, 3)
  line L33 (33, 3) -> (33, 0)
  line L34 (33, 0) -> (43, 0)
  line L35 (43, 0) -> (43, 3)
  line L36 (43, 3) -> (53, 3)
  line L37 (53, 3) -> (53, 0)
  line L38 (53, 0) -> (63, 0)
  line L39 (63, 0) -> (63, 3)
  line L40 (63, 3) -> (73, 3)
  line L41 (73, 3) -> (73, 0)
  line L42 (73, 0) -> (76, 0)
  line L43 (76, 0) -> (76, 13)
  line L44 (76, 13) -> (73, 13)
  line L45 (73, 13) -> (73, 23)
  line L46 (73, 23) -> (76, 23)
  line L47 (76, 23) -> (76, 33)
  line L48 (76, 33) -> (73, 33)
  line L49 (73, 33) -> (73, 43)
  line L50 (73, 43) -> (76, 43)
  line L51 (76, 43) -> (76, 56)
  line L52 (76, 56) -> (73, 56)
  line L53 (73, 56) -> (73, 53)
  line L54 (73, 53) -> (63, 53)
  line L55 (63, 53) -> (63, 56)
  line L56 (15.4286, 11.2562) -> (61.3514, 11.2562) construction
  line L57 (61.3514, 11.2562) -> (61.3514, 26.2562) construction
  line L58 (61.3514, 26.2562) -> (15.4286, 26.2562) construction
  line L59 (15.4286, 26.2562) -> (15.4286, 11.2562) construction
  text T0 "HeLL0!" font "Arial" height 15 align ink ink in box 0 x 0 at (15.4386, 11.2762) x (1, 0) y (0, 1) spacing 1 height is em
  constraint perpendicular L56 L57
  constraint parallel L56 L58
  constraint parallel L57 L59
extrude "Extrude5" cut sketch "Sketch5" against normal blind 1 text T0 bodies 2
sketch "Sketch6" plane through (0, 76, 0) normal (0, 1, 0) x (-1, 0, 0)
  line L0 (183, 0) -> (193, 0)
  line L1 (193, 0) -> (193, 13)
  line L2 (193, 13) -> (196, 13)
  line L3 (196, 13) -> (196, 23)
  line L4 (196, 23) -> (193, 23)
  line L5 (193, 23) -> (193, 33)
  line L6 (193, 33) -> (196, 33)
  line L7 (196, 33) -> (196, 43)
  line L8 (196, 43) -> (193, 43)
  line L9 (193, 43) -> (193, 56)
  line L10 (193, 56) -> (183, 56)
  line L11 (183, 56) -> (183, 53)
  line L12 (183, 53) -> (173, 53)
  line L13 (173, 53) -> (173, 56)
  line L14 (173, 56) -> (163, 56)
  line L15 (163, 56) -> (163, 53)
  line L16 (163, 53) -> (153, 53)
  line L17 (153, 53) -> (153, 56)
  line L18 (153, 56) -> (143, 56)
  line L19 (143, 56) -> (143, 53)
  line L20 (143, 53) -> (133, 53)
  line L21 (133, 53) -> (133, 56)
  line L22 (133, 56) -> (123, 56)
  line L23 (123, 56) -> (123, 53)
  line L24 (123, 53) -> (113, 53)
  line L25 (113, 53) -> (113, 56)
  line L26 (113, 56) -> (103, 56)
  line L27 (103, 56) -> (103, 53)
  line L28 (103, 53) -> (93, 53)
  line L29 (93, 53) -> (93, 56)
  line L30 (93, 56) -> (83, 56)
  line L31 (83, 56) -> (83, 53)
  line L32 (83, 53) -> (73, 53)
  line L33 (73, 53) -> (73, 56)
  line L34 (73, 56) -> (63, 56)
  line L35 (63, 56) -> (63, 53)
  line L36 (63, 53) -> (53, 53)
  line L37 (53, 53) -> (53, 56)
  line L38 (53, 56) -> (43, 56)
  line L39 (43, 56) -> (43, 53)
  line L40 (43, 53) -> (33, 53)
  line L41 (33, 53) -> (33, 56)
  line L42 (33, 56) -> (23, 56)
  line L43 (23, 56) -> (23, 53)
  line L44 (23, 53) -> (13, 53)
  line L45 (13, 53) -> (13, 56)
  line L46 (13, 56) -> (3, 56)
  line L47 (3, 56) -> (3, 43)
  line L48 (3, 43) -> (0, 43)
  line L49 (0, 43) -> (0, 33)
  line L50 (0, 33) -> (3, 33)
  line L51 (3, 33) -> (3, 23)
  line L52 (3, 23) -> (0, 23)
  line L53 (0, 23) -> (0, 13)
  line L54 (0, 13) -> (3, 13)
  line L55 (3, 13) -> (3, 0)
  line L56 (3, 0) -> (13, 0)
  line L57 (13, 0) -> (13, 3)
  line L58 (13, 3) -> (23, 3)
  line L59 (23, 3) -> (23, 0)
  line L60 (23, 0) -> (33, 0)
  line L61 (33, 0) -> (33, 3)
  line L62 (33, 3) -> (43, 3)
  line L63 (43, 3) -> (43, 0)
  line L64 (43, 0) -> (53, 0)
  line L65 (53, 0) -> (53, 3)
  line L66 (53, 3) -> (63, 3)
  line L67 (63, 3) -> (63, 0)
  line L68 (63, 0) -> (73, 0)
  line L69 (73, 0) -> (73, 3)
  line L70 (73, 3) -> (83, 3)
  line L71 (83, 3) -> (83, 0)
  line L72 (83, 0) -> (93, 0)
  line L73 (93, 0) -> (93, 3)
  line L74 (93, 3) -> (103, 3)
  line L75 (103, 3) -> (103, 0)
  line L76 (103, 0) -> (113, 0)
  line L77 (113, 0) -> (113, 3)
  line L78 (113, 3) -> (123, 3)
  line L79 (123, 3) -> (123, 0)
  line L80 (123, 0) -> (133, 0)
  line L81 (133, 0) -> (133, 3)
  line L82 (133, 3) -> (143, 3)
  line L83 (143, 3) -> (143, 0)
  line L84 (143, 0) -> (153, 0)
  line L85 (153, 0) -> (153, 3)
  line L86 (153, 3) -> (163, 3)
  line L87 (163, 3) -> (163, 0)
  line L88 (163, 0) -> (173, 0)
  line L89 (173, 0) -> (173, 3)
  line L90 (173, 3) -> (183, 3)
  line L91 (183, 3) -> (183, 0)
  line L92 (0, 0) -> (10, 0)
  line L93 (10, 0) -> (10, 15)
  line L94 (10, 15) -> (95, 15)
  line L95 (95, 15) -> (95, 18)
  line L96 (95, 18) -> (10, 18)
  line L97 (10, 18) -> (10, 15)
  line L98 (180, 50) -> (187, 50)
  line L99 (187, 50) -> (187, 49)
  line L100 (187, 49) -> (180, 49)
  line L101 (180, 49) -> (180, 50)
  line L102 (95, 18) -> (95, 33)
  line L103 (95, 33) -> (115, 33)
  line L104 (115, 33) -> (186, 33)
  line L105 (186, 33) -> (186, 36)
  line L106 (186, 36) -> (115, 36)
  line L107 (115, 36) -> (115, 33)
  dimension "d145" = 10
  dimension "d146" = 15
  dimension "d147" = 85
  dimension "d148" = 3
  dimension "d149" = 7
  dimension "d150" = 1
  dimension "d162" = 15
  dimension "d163" = 20
  dimension "d164" = 71
  dimension "d165" = 3
  constraint coincident L92.start origin
  constraint perpendicular L55 L92
  constraint perpendicular L62 L93
  constraint horizontal L94
  constraint vertical L95
  constraint horizontal L96
  constraint vertical L97
  constraint horizontal L98
  constraint vertical L99
  constraint horizontal L100
  constraint vertical L101
  constraint perpendicular L96 L102
  constraint perpendicular L95 L103
  constraint horizontal L104
  constraint vertical L105
  constraint horizontal L106
  constraint vertical L107
  measures "d145" distance of L92.start L92.end
  measures "d146" distance of L92.end L93.end
  measures "d147" distance of L93.end L94.end
  measures "d148" distance of L93.end L96.end
  measures "d149" distance of L98.start L98.end
  measures "d150" distance of L98.start L100.end
  measures "d162" distance of L95.end L102.end
  measures "d163" distance of L102.end L103.end
  measures "d164" distance of L103.end L104.end
  measures "d165" distance of L103.end L106.end
extrude "Extrude9" cut sketch "Sketch6" against normal blind 76 contours L94 L95 L96 L97 | L98 L99 L100 L101 | L104 L105 L106 L107 bodies 3 5
extrude "Extrude8" cut sketch "Sketch6" against normal blind 76 contours L94 L95 L96 L97 | L98 L99 L100 L101 bodies 3 5
extrude "Extrude6" cut sketch "Sketch6" against normal blind 3 contours L94 L95 L96 L97 | L98 L99 L100 L101 bodies 3
sketch "Sketch7" plane through (0, 0, 56) normal (0, 0, 1) x (-1, 0, 0)
  line L0 (13, -3) -> (0, -3)
  line L1 (0, -3) -> (0, -13)
  line L2 (0, -13) -> (3, -13)
  line L3 (3, -13) -> (3, -23)
  line L4 (3, -23) -> (0, -23)
  line L5 (0, -23) -> (0, -33)
  line L6 (0, -33) -> (3, -33)
  line L7 (3, -33) -> (3, -43)
  line L8 (3, -43) -> (0, -43)
  line L9 (0, -43) -> (0, -53)
  line L10 (0, -53) -> (3, -53)
  line L11 (3, -53) -> (3, -63)
  line L12 (3, -63) -> (0, -63)
  line L13 (0, -63) -> (0, -73)
  line L14 (0, -73) -> (13, -73)
  line L15 (13, -73) -> (13, -76)
  line L16 (13, -76) -> (23, -76)
  line L17 (23, -76) -> (23, -73)
  line L18 (23, -73) -> (33, -73)
  line L19 (33, -73) -> (33, -76)
  line L20 (33, -76) -> (43, -76)
  line L21 (43, -76) -> (43, -73)
  line L22 (43, -73) -> (53, -73)
  line L23 (53, -73) -> (53, -76)
  line L24 (53, -76) -> (63, -76)
  line L25 (63, -76) -> (63, -73)
  line L26 (63, -73) -> (73, -73)
  line L27 (73, -73) -> (73, -76)
  line L28 (73, -76) -> (83, -76)
  line L29 (83, -76) -> (83, -73)
  line L30 (83, -73) -> (93, -73)
  line L31 (93, -73) -> (93, -76)
  line L32 (93, -76) -> (103, -76)
  line L33 (103, -76) -> (103, -73)
  line L34 (103, -73) -> (113, -73)
  line L35 (113, -73) -> (113, -76)
  line L36 (113, -76) -> (123, -76)
  line L37 (123, -76) -> (123, -73)
  line L38 (123, -73) -> (133, -73)
  line L39 (133, -73) -> (133, -76)
  line L40 (133, -76) -> (143, -76)
  line L41 (143, -76) -> (143, -73)
  line L42 (143, -73) -> (153, -73)
  line L43 (153, -73) -> (153, -76)
  line L44 (153, -76) -> (163, -76)
  line L45 (163, -76) -> (163, -73)
  line L46 (163, -73) -> (173, -73)
  line L47 (173, -73) -> (173, -76)
  line L48 (173, -76) -> (183, -76)
  line L49 (183, -76) -> (183, -73)
  line L50 (183, -73) -> (196, -73)
  line L51 (196, -73) -> (196, -63)
  line L52 (196, -63) -> (193, -63)
  line L53 (193, -63) -> (193, -53)
  line L54 (193, -53) -> (196, -53)
  line L55 (196, -53) -> (196, -43)
  line L56 (196, -43) -> (193, -43)
  line L57 (193, -43) -> (193, -33)
  line L58 (193, -33) -> (196, -33)
  line L59 (196, -33) -> (196, -23)
  line L60 (196, -23) -> (193, -23)
  line L61 (193, -23) -> (193, -13)
  line L62 (193, -13) -> (196, -13)
  line L63 (196, -13) -> (196, -3)
  line L64 (196, -3) -> (183, -3)
  line L65 (183, -3) -> (183, 0)
  line L66 (183, 0) -> (173, 0)
  line L67 (173, 0) -> (173, -3)
  line L68 (173, -3) -> (163, -3)
  line L69 (163, -3) -> (163, 0)
  line L70 (163, 0) -> (153, 0)
  line L71 (153, 0) -> (153, -3)
  line L72 (153, -3) -> (143, -3)
  line L73 (143, -3) -> (143, 0)
  line L74 (143, 0) -> (133, 0)
  line L75 (133, 0) -> (133, -3)
  line L76 (133, -3) -> (123, -3)
  line L77 (123, -3) -> (123, 0)
  line L78 (123, 0) -> (113, 0)
  line L79 (113, 0) -> (113, -3)
  line L80 (113, -3) -> (103, -3)
  line L81 (103, -3) -> (103, 0)
  line L82 (103, 0) -> (93, 0)
  line L83 (93, 0) -> (93, -3)
  line L84 (93, -3) -> (83, -3)
  line L85 (83, -3) -> (83, 0)
  line L86 (83, 0) -> (73, 0)
  line L87 (73, 0) -> (73, -3)
  line L88 (73, -3) -> (63, -3)
  line L89 (63, -3) -> (63, 0)
  line L90 (63, 0) -> (53, 0)
  line L91 (53, 0) -> (53, -3)
  line L92 (53, -3) -> (43, -3)
  line L93 (43, -3) -> (43, 0)
  line L94 (43, 0) -> (33, 0)
  line L95 (33, 0) -> (33, -3)
  line L96 (33, -3) -> (23, -3)
  line L97 (23, -3) -> (23, 0)
  line L98 (23, 0) -> (13, 0)
  line L99 (13, 0) -> (13, -3)
  line L100 (8.8818, -6.8746) -> (7.3818, -6.8746)
  line L101 (7.3818, -6.8746) -> (7.3818, -12.8746)
  line L102 (7.3818, -12.8746) -> (8.8818, -12.8746)
  line L103 (8.8818, -12.8746) -> (8.8818, -6.8746)
  line L104 (0, -75) -> (0, -68)
  line L105 (0, -68) -> (90, -68)
  line L106 (90, -68) -> (32, -68)
  line L107 (32, -68) -> (32, -48)
  line L108 (32, -48) -> (90, -48)
  line L109 (90, -48) -> (90, -68)
  dimension "d153" = 1.5
  dimension "d154" = 6
  dimension "d155" = 90
  dimension "d156" = 58
  dimension "d157" = 20
  constraint horizontal L100
  constraint vertical L101
  constraint horizontal L102
  constraint vertical L103
  constraint midpoint L13 L104.end
  constraint perpendicular L14 L104
  constraint perpendicular L13 L105
  constraint horizontal L106
  constraint vertical L107
  constraint horizontal L108
  constraint vertical L109
  measures "d153" distance of L100.start L100.end
  measures "d154" distance of L100.start L102.end
  measures "d155" distance of L104.end L105.end
  measures "d156" distance of L105.end L106.end
  measures "d157" distance of L105.end L108.end
extrude "Extrude7" cut sketch "Sketch7" against normal blind 3 contours L100 L101 L102 L103 | L105 L106 L107 L108 L109 bodies 6